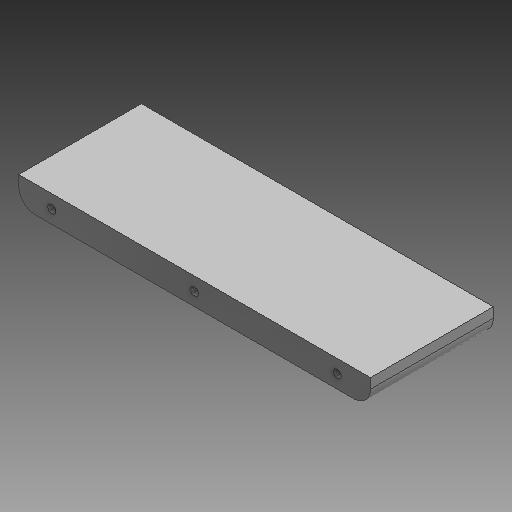
# Autodesk Inventor part: side 2
Saved by Autodesk Inventor 2019 (Build 230136000, 136)
## iProperties
Created: 2018-05-03
Part Number: side 2
Material: Aluminum 6061
Document SubType Name: Modeling
Designer: SimonD
Density: 2.7 g/cm^3
Appearance: Aluminum - Polished
Author: SimonD
Autodesk Inventor part; units mm, degrees
ref_plane "YZ Plane" through (0, 0, 0) normal (1, 0, 0) x (0, 1, 0)
ref_plane "XZ Plane" through (0, 0, 0) normal (0, 1, 0) x (-1, 0, 0)
ref_plane "XY Plane" through (0, 0, 0) normal (0, 0, 1) x (1, 0, 0)
sketch "Sketch1" plane through (0, 0, 0) normal (0, 0, 1) x (1, 0, 0)
  line L0 (-53, 4) -> (53, 4)
  line L1 (53, 4) -> (53, -4)
  line L2 (53, -4) -> (-53, -4)
  line L3 (-53, -4) -> (-53, 4)
  line L4 (-53, 4) -> (53, -4) construction
  line L5 (53, 4) -> (-53, -4) construction
  point P0 (0, 0)
  dimension "d0" = 106
  dimension "d1" = 8
  constraints: 12 end point, 2 midpoint, 2 parallel, 1 horizontal, 1 perpendicular
  measures "d0" distance of L1.end L2.end
  measures "d1" distance between parallel lines of L2 L0
extrude "Extrusion1" add sketch "Sketch1" along normal blind 37
sketch "Sketch2" plane through (0, 0, 37) normal (0, 0, 1) x (1, 0, 0)
  line L0 (-53, 4) -> (-53, -4) projected
  line L1 (53, -4) -> (53, 4) projected
  point P0 (0, 0)
  point P1 (-43, 0)
  point P2 (0, 0)
  point P3 (43, 0)
  dimension "d4" = 10
  dimension "d5" = 10
  constraints: 1 coincident
  measures "d4" distance from line of point (-43, 0) L0
  measures "d5" distance from line of L1 point (43, 0)
hole "Hole1" at (-43, 0, 37) at (0, 0, 37) at (43, 0, 37) direction (0, 0, -1) diameter 2.459 depth 8 tip angle 118 thread size "M3x0.5" class "6H" standard "ISO Metric profile"
sketch "Sketch3" plane through (0, 0, 0) normal (0, 0, -1) x (-1, 0, 0)
  circle A0 centre (43, 0) radius 1.2295 projected
  circle A1 centre (0, 0) radius 1.2295 projected
  circle A2 centre (-43, 0) radius 1.2295 projected
  constraints: 3 coincident
hole "Hole2" at (-43, 0, 0) at (0, 0, 0) at (43, 0, 0) direction (0, 0, 1) diameter 2.459 depth 8.8 tip angle 118 thread size "M3x0.5" class "6H" standard "ISO Metric profile"
fillet "Fillet1" radius 5 2 edges at (-53, -4, 18.5) (53, -4, 18.5)
sketch "Sketch4" plane through (0, 0, 37) normal (0, 0, 1) x (1, 0, 0)
  point P0 (0, 0)
  point P1 (-25, 0)
  point P2 (25, 0)
  dimension "d21" = 25
  dimension "d22" = 25
  measures "d21" distance of point (-25, 0) point (0, 0)
  measures "d22" distance of point (25, 0) point (0, 0)
hole "Hole3" [suppressed]
sketch "Sketch5" plane through (0, 0, 0) normal (0, 0, -1) x (-1, 0, 0)
  circle A0 centre (25, 0) radius 1.5 projected
  circle A1 centre (-25, 0) radius 1.5 projected
  point P0 (0, 0)
  constraints: 2 coincident
hole "Hole4" [suppressed]
body "Solid1"
